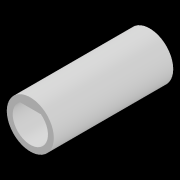
# Autodesk Inventor part: ForearmShaftLock
Saved by Autodesk Inventor 2020 (Build 240168000, 168)
## iProperties
Created: 2021-01-24
Part Number: ForearmShaftLock
Material: Generic
Document SubType Name: Modeling
Designer: valer
Density: 1 g/cm^3
Appearance: Default
Author: valer
Autodesk Inventor part; units mm, degrees
ref_plane "YZ Plane" through (0, 0, 0) normal (1, 0, 0) x (0, 1, 0)
ref_plane "XZ Plane" through (0, 0, 0) normal (0, 1, 0) x (-1, 0, 0)
ref_plane "XY Plane" through (0, 0, 0) normal (0, 0, 1) x (1, 0, 0)
sketch "Sketch1" plane through (0, 0, 0) normal (0, 0, 1) x (1, 0, 0)
  circle A0 centre (0, 0) radius 3
  line L0 (0, -3) -> (0, 0)
  line L1 (-1.8, 2.4) -> (1.8, 2.4)
  circle A1 centre (0, 0) radius 4
  dimension "d0" = 6
  dimension "d1" = 5.4
  dimension "d2" = 8
  constraints: 4 end point, 3 point on circle, 2 centre point, 2 coincident, 1 horizontal, 1 vertical
  measures "d0" diameter of A0
  measures "d1" distance from line of L0.start L1
  measures "d2" diameter of A1
extrude "Extrusion1" add sketch "Sketch1" along normal blind 20.32 contours L1 A0 | A1 picked at (0, 2.6)
body "Solid1"
